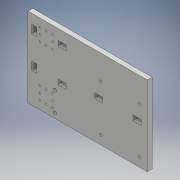
# Autodesk Inventor part: base
Saved by Autodesk Inventor 2017 (Build 210142000, 142)
## iProperties
Part Number: base
Material: Générique
Document SubType Name: Modeling
Designer: Thomas
Density: 1 g/cm^3
Appearance: Par défaut
Author: Thomas
Autodesk Inventor part; units mm, degrees
ref_plane "YZ Plane" through (0, 0, 0) normal (1, 0, 0) x (0, 1, 0)
ref_plane "XZ Plane" through (0, 0, 0) normal (0, 1, 0) x (-1, 0, 0)
ref_plane "XY Plane" through (0, 0, 0) normal (0, 0, 1) x (1, 0, 0)
sketch "Esquisse1" plane through (0, 0, 0) normal (0, 1, 0) x (-1, 0, 0)
  line L0 (-75, 50) -> (75, 50)
  line L1 (75, 50) -> (75, -50)
  line L2 (75, -50) -> (-75, -50)
  line L3 (-75, -50) -> (-75, 50)
  line L4 (75, 50) -> (-75, -50) construction
  circle A0 centre (60, -40) radius 1.05
  circle A1 centre (52, -40) radius 1.05
  circle A2 centre (44, -40) radius 1.05
  circle A3 centre (60, -32) radius 1.05
  circle A4 centre (52, -32) radius 1.05 construction
  circle A5 centre (44, -32) radius 1.05
  circle A6 centre (60, -24) radius 1.05
  circle A7 centre (52, -24) radius 1.05
  circle A8 centre (44, -24) radius 1.05
  line L5 (75, 0) -> (-75, 0) construction
  circle A9 centre (60, 40) radius 1.05
  circle A10 centre (52, 40) radius 1.05
  circle A11 centre (44, 40) radius 1.05
  circle A12 centre (60, 32) radius 1.05
  circle A13 centre (52, 32) radius 1.05 construction
  circle A14 centre (44, 32) radius 1.05
  circle A15 centre (60, 24) radius 1.05
  circle A16 centre (52, 24) radius 1.05
  circle A17 centre (44, 24) radius 1.05
  line L6 (64, -2.0284) -> (70, -2.0284)
  line L7 (70, -2.0284) -> (70, -12.0284)
  line L8 (70, -12.0284) -> (64, -12.0284)
  line L9 (64, -12.0284) -> (64, -2.0284)
  line L10 (64, -2.0284) -> (70, -12.0284) construction
  line L11 (70, -2.0284) -> (64, -12.0284) construction
  line L12 (64, 37.9716) -> (70, 37.9716)
  line L13 (70, 37.9716) -> (70, 27.9716)
  line L14 (70, 27.9716) -> (64, 27.9716)
  line L15 (64, 27.9716) -> (64, 37.9716)
  line L16 (64, 37.9716) -> (70, 27.9716) construction
  line L17 (70, 37.9716) -> (64, 27.9716) construction
  line L18 (27, -5.0284) -> (37, -5.0284)
  line L19 (37, -5.0284) -> (37, -11.0284)
  line L20 (37, -11.0284) -> (27, -11.0284)
  line L21 (27, -11.0284) -> (27, -5.0284)
  line L22 (27, -5.0284) -> (37, -11.0284) construction
  line L23 (37, -5.0284) -> (27, -11.0284) construction
  line L24 (27, 36.9716) -> (37, 36.9716)
  line L25 (37, 36.9716) -> (37, 30.9716)
  line L26 (37, 30.9716) -> (27, 30.9716)
  line L27 (27, 30.9716) -> (27, 36.9716)
  line L28 (27, 36.9716) -> (37, 30.9716) construction
  line L29 (37, 36.9716) -> (27, 30.9716) construction
  point P0 (0, 0)
  point P1 (67, -7.0284)
  point P2 (67, 32.9716)
  point P3 (32, -8.0284)
  point P4 (32, 33.9716)
  dimension "d0" = 150
  dimension "d1" = 100
  dimension "d2" = 2.1
  dimension "d3" = 10
  dimension "d4" = 15
  dimension "d7" = 8
  dimension "d10" = 8
  dimension "d25" = 50
  dimension "d26" = 0
  dimension "d27" = 6
  dimension "d28" = 10
  dimension "d29" = 6
  dimension "d30" = 10
  dimension "d31" = 50
  dimension "d32" = 5
  dimension "d33" = 5
  dimension "d34" = 10
  dimension "d35" = 6
  dimension "d36" = 6
  dimension "d37" = 36
  dimension "d38" = 35
  dimension "d39" = 1
  constraints: 60 end point, 18 centre point, 11 midpoint, 10 parallel, 9 symmetric about line, 6 horizontal, 5 perpendicular, 1 point on line, 1 vertical, 25 other
  measures "d0" distance of L1.end L2.end
  measures "d1" distance of L0.end L1.end
  measures "d2" diameter of A0
  measures "d3" distance from line of L2 A0.centre
  measures "d4" distance from line of L1 A0.centre
  measures "d7" distance of A0.centre A1.centre
  measures "d10" distance of A0.centre A3.centre
  measures "d25" distance between parallel lines of L2 L5
  measures "d26" distance from line of point (0, 0) L5
  measures "d27" distance of L7.end L8.end
  measures "d28" distance of L6.end L7.end
  measures "d29" distance of L13.end L14.end
  measures "d30" distance of L12.end L13.end
  measures "d31" distance between parallel lines of L12 L8
  measures "d32" distance between parallel lines of L1 L7
  measures "d33" distance between parallel lines of L1 L13
  measures "d34" distance of L19.end L20.end
  measures "d35" distance of L18.end L19.end
  measures "d36" distance of L24.end L25.end
  measures "d37" distance between parallel lines of L26 L18
  measures "d38" horizontal distance of point (67, -7.028) point (32, -8.028)
  measures "d39" distance between parallel lines of L24 L12
ref_plane "Plan de construction1" through (0, 6, 0) normal (0, 1, 0) x (1, 0, 0)
extrude "Extrusion2" add sketch "Esquisse1" along normal blind 6
sketch "Esquisse3" plane through (0, 6, 0) normal (0, 1, 0) x (1, 0, 0)
  line L0 (-37, -36.9716) -> (-37, -30.9716) construction
  line L1 (-37, -30.9716) -> (-27, -30.9716) construction
  line L2 (-27, -30.9716) -> (-27, -36.9716) construction
  line L3 (-27, -36.9716) -> (-37, -36.9716) construction
  line L4 (-37, 5.0284) -> (-37, 11.0284) construction
  line L5 (-37, 11.0284) -> (-27, 11.0284) construction
  line L6 (-27, 11.0284) -> (-27, 5.0284) construction
  line L7 (-27, 5.0284) -> (-37, 5.0284) construction
  line L8 (-70, -37.9716) -> (-70, -27.9716) construction
  line L9 (-70, -27.9716) -> (-64, -27.9716) construction
  line L10 (-64, -27.9716) -> (-64, -37.9716) construction
  line L11 (-64, -37.9716) -> (-70, -37.9716) construction
  line L12 (-70, 2.0284) -> (-70, 12.0284) construction
  line L13 (-70, 12.0284) -> (-64, 12.0284) construction
  line L14 (-64, 12.0284) -> (-64, 2.0284) construction
  line L15 (-64, 2.0284) -> (-70, 2.0284) construction
  circle A0 centre (-60, -40) radius 1.05 construction
  circle A1 centre (-44, -24) radius 1.05 construction
  circle A2 centre (-44, -32) radius 1.05 construction
  circle A3 centre (-44, -40) radius 1.05 construction
  circle A4 centre (-52, -24) radius 1.05 construction
  circle A5 centre (-52, -40) radius 1.05 construction
  circle A6 centre (-60, -24) radius 1.05 construction
  circle A7 centre (-60, -32) radius 1.05 construction
  circle A8 centre (-44, 24) radius 1.05 construction
  circle A9 centre (-52, 24) radius 1.05 construction
  circle A10 centre (-60, 24) radius 1.05 construction
  circle A11 centre (-44, 32) radius 1.05 construction
  circle A12 centre (-60, 32) radius 1.05 construction
  circle A13 centre (-44, 40) radius 1.05 construction
  circle A14 centre (-52, 40) radius 1.05 construction
  circle A15 centre (-60, 40) radius 1.05 construction
  line L16 (-75, -50) -> (75, -50) construction
  line L17 (75, -50) -> (75, 50) construction
  line L18 (75, 50) -> (-75, 50) construction
  line L19 (-75, 50) -> (-75, -50) construction
  line L20 (-27, 8.0284) -> (13, 8.0284) construction
  line L21 (69, -42.5) -> (13, -42.5) construction
  line L22 (13, -42.5) -> (13, 42.5) construction
  line L23 (13, 42.5) -> (69, 42.5) construction
  line L24 (69, 42.5) -> (69, -42.5) construction
  line L25 (69, -42.5) -> (13, 42.5) construction
  line L26 (13, -42.5) -> (69, 42.5) construction
  circle A16 centre (16.75, 38.75) radius 1.5
  circle A17 centre (65.75, 38.75) radius 1.5
  circle A18 centre (16.75, -19.25) radius 1.5
  circle A19 centre (65.75, -19.25) radius 1.5
  point P0 (0, 0)
  point P1 (41, 0)
  dimension "d42" = 40
  dimension "d43" = 56
  dimension "d44" = 85
  dimension "d45" = 0
  dimension "d46" = 3
  dimension "d47" = 3.75
  dimension "d48" = 3.75
  dimension "d51" = 49
  dimension "d54" = 58
  constraints: 14 end point, 4 centre point, 3 horizontal, 3 midpoint, 2 parallel, 1 perpendicular, 1 vertical, 6 other
  measures "d42" distance of L20.start L20.end
  measures "d43" distance of L22.end L23.end
  measures "d44" distance of L21.end L22.end
  measures "d45" distance from line of L22 L20.end
  measures "d46" diameter of A16
  measures "d47" distance from line of L23 A16.centre
  measures "d48" distance from line of L22 A16.centre
  measures "d51" distance of A16.centre A17.centre
  measures "d54" distance of A16.centre A18.centre
extrude "Extrusion3" cut sketch "Esquisse3" against normal blind 6
sketch "Esquisse4" plane through (0, 6, 0) normal (0, 1, 0) x (1, 0, 0)
  line L0 (-40.9885, 18.973) -> (-1.9885, 18.973) construction
  line L1 (-1.9885, 18.973) -> (-1.9885, 43.973) construction
  line L2 (-1.9885, 43.973) -> (-40.9885, 43.973) construction
  line L3 (-40.9885, 43.973) -> (-40.9885, 18.973) construction
  line L4 (-40.9885, 18.973) -> (-1.9885, 43.973) construction
  line L5 (-1.9885, 18.973) -> (-40.9885, 43.973) construction
  circle A0 centre (-40.9885, 43.973) radius 2
  circle A1 centre (-40.9885, 18.973) radius 2
  point P0 (0, 0)
  point P1 (-21.4885, 31.473)
  dimension "d59" = 39
  dimension "d60" = 25
  dimension "d61" = 4
  dimension "d62" = 4
  constraints: 12 end point, 2 centre point, 2 coincident, 2 midpoint, 2 parallel, 1 horizontal, 1 perpendicular
  measures "d59" distance of L2.end L1.end
  measures "d60" distance of L1.end L0.end
  measures "d61" diameter of A0
  measures "d62" diameter of A1
extrude "Extrusion4" cut sketch "Esquisse4" against normal blind 10
sketch "Esquisse5" plane through (0, 6, 0) normal (0, 1, 0) x (1, 0, 0)
  line L0 (8.9522, -3) -> (18.9522, -3)
  line L1 (18.9522, -3) -> (18.9522, 3)
  line L2 (18.9522, 3) -> (8.9522, 3)
  line L3 (8.9522, 3) -> (8.9522, -3)
  line L4 (8.9522, -3) -> (18.9522, 3) construction
  line L5 (18.9522, -3) -> (8.9522, 3) construction
  line L6 (57.3085, -3) -> (67.3085, -3)
  line L7 (67.3085, -3) -> (67.3085, 3)
  line L8 (67.3085, 3) -> (57.3085, 3)
  line L9 (57.3085, 3) -> (57.3085, -3)
  line L10 (57.3085, -3) -> (67.3085, 3) construction
  line L11 (67.3085, -3) -> (57.3085, 3) construction
  point P0 (0, 0)
  point P1 (13.9522, 0)
  point P2 (62.3085, 0)
  dimension "d65" = 10
  dimension "d66" = 6
  dimension "d67" = 10
  dimension "d68" = 6
  constraints: 24 end point, 4 midpoint, 4 parallel, 2 horizontal, 2 perpendicular
  measures "d65" distance of L2.end L1.end
  measures "d66" distance of L1.end L0.end
  measures "d67" distance of L8.end L7.end
  measures "d68" distance of L7.end L6.end
extrude "Extrusion5" cut sketch "Esquisse5" against normal blind 10
